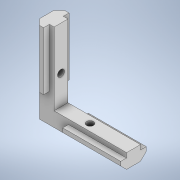
# Autodesk Inventor part: Equerre
Saved by Autodesk Inventor 2020 (Build 240168000, 168)
## iProperties
Created: 2019-11-28
Part Number: Equerre
Material: Générique
Document SubType Name: Modeling
Designer: erwan
Density: 1 g/cm^3
Appearance: Par défaut
Author: erwan
Autodesk Inventor part; units mm, degrees
ref_plane "YZ Plane" through (0, 0, 0) normal (1, 0, 0) x (0, 1, 0)
ref_plane "XZ Plane" through (0, 0, 0) normal (0, 1, 0) x (-1, 0, 0)
ref_plane "XY Plane" through (0, 0, 0) normal (0, 0, 1) x (1, 0, 0)
sketch "Esquisse1" plane through (0, 0, 0) normal (0, 1, 0) x (-1, 0, 0)
  line L0 (2.125, 0) -> (2.125, 3)
  line L1 (2.125, 0) -> (2.125, -3)
  line L2 (-2.125, 5.5) -> (-0.375, 5.5)
  line L3 (2.125, 3) -> (-0.375, 5.5)
  line L4 (-2.125, -5.5) -> (-0.375, -5.5)
  line L5 (-0.375, -5.5) -> (2.125, -3)
  line L6 (-2.125, 3) -> (-4.125, 3)
  line L7 (-4.125, 3) -> (-4.125, -3)
  line L8 (-4.125, -3) -> (-2.125, -3)
  line L9 (-2.125, 5.5) -> (-2.125, 3)
  line L10 (-2.125, -3) -> (-2.125, -5.5)
  point P0 (0, 0)
  dimension "d2" = 3
  dimension "d3" = 3
  dimension "d4" = 1.75
  dimension "d5" = 1.75
  dimension "d6" = 2
  constraints: 22 end point, 2 equal length, 1 horizontal, 1 perpendicular, 1 vertical
  measures "d2" distance of L0.start L0.end
  measures "d3" distance of L0.start L1.end
  measures "d4" distance of L2.start L2.end
  measures "d5" distance of L4.start L4.end
  measures "d6" distance of L8.end L7.end
extrude "Extrusion1" add sketch "Esquisse1" along normal blind 25
sketch "Esquisse2" plane through (0, 0, 0) normal (0, -1, 0) x (1, 0, 0)
  line L0 (-2.125, -3) -> (-2.125, 3) projected
  line L1 (2.125, 3) -> (4.125, 3) projected
  line L2 (-2.125, 3) -> (4.125, 3)
  line L3 (4.125, 3) -> (4.125, -3)
  line L4 (4.125, -3) -> (-2.125, -3)
  line L5 (-2.125, -3) -> (-2.125, 3)
  point P0 (0, 0)
  constraints: 8 end point, 2 parallel, 1 collinear, 1 perpendicular
extrude "Extrusion2" add sketch "Esquisse2" along normal blind 12.5
sketch "Esquisse3" plane through (4.125, 25, 3) normal (1, 0, 0) x (0, 0, -1)
  line L0 (0, -25) -> (0, -37.5) projected
  line L1 (6, -25) -> (6, -37.5) projected
  line L2 (0, -37.5) -> (6, -37.5)
  line L3 (6, -37.5) -> (6, -31.25)
  line L4 (6, -31.25) -> (0, -31.25)
  line L5 (0, -31.25) -> (0, -37.5)
  point P0 (3, -25)
  point P1 (0, -31.25)
  dimension "d11" = 6.25
  constraints: 8 end point, 2 parallel, 1 horizontal, 1 midpoint, 1 perpendicular
  measures "d11" distance of L3.end L2.end
extrude "Extrusion3" add sketch "Esquisse3" along normal blind 6.25
sketch "Esquisse4" plane through (10.375, 25, 3) normal (1, 0, 0) x (0, 0, -1)
  line L0 (6, -31.25) -> (0, -31.25) projected
  line L1 (0, -31.25) -> (0, -33.25)
  line L2 (0, -33.25) -> (-2.5, -33.25)
  line L3 (-2.5, -33.25) -> (-2.5, -35)
  line L4 (-2.5, -35) -> (0, -37.5)
  line L5 (6, -31.25) -> (6, -33.25)
  line L6 (6, -33.25) -> (8.5, -33.25)
  line L7 (8.5, -33.25) -> (8.5, -35)
  line L8 (8.5, -35) -> (6, -37.5)
  line L9 (6, -31.25) -> (0, -31.25)
  line L10 (0, -37.5) -> (6, -37.5) projected
  line L11 (0, -37.5) -> (6, -37.5)
  dimension "d14" = 2
  dimension "d15" = 2.5
  dimension "d16" = 1.75
  dimension "d17" = 2
  dimension "d18" = 2.5
  dimension "d19" = 1.75
  constraints: 20 end point, 3 perpendicular, 2 horizontal, 1 point on line
  measures "d14" distance of L0.end L1.end
  measures "d15" distance of L1.end L2.end
  measures "d16" distance of L2.end L3.end
  measures "d17" distance of L5.start L5.end
  measures "d18" distance of L5.end L6.end
  measures "d19" distance of L6.end L7.end
extrude "Extrusion4" add sketch "Esquisse4" along normal blind 25
sketch "Esquisse6" plane through (0, -12.5, 0) normal (0, -1, 0) x (1, 0, 0)
  circle A0 centre (16.625, 0) radius 1.5
  point P0 (0, 0)
  dimension "d22" = 3
  constraints: 1 centre point
  measures "d22" diameter of A0
extrude "Extrusion5" cut sketch "Esquisse6" against normal blind 25
sketch "Esquisse7" plane through (-2.125, 0, 3) normal (-1, 0, 0) x (0, 0, 1)
  circle A0 centre (-3, 6.25) radius 1.5
  point P0 (-3, 0)
  dimension "d25" = 3
  constraints: 1 centre point
  measures "d25" diameter of A0
extrude "Extrusion6" cut sketch "Esquisse7" against normal blind 25
